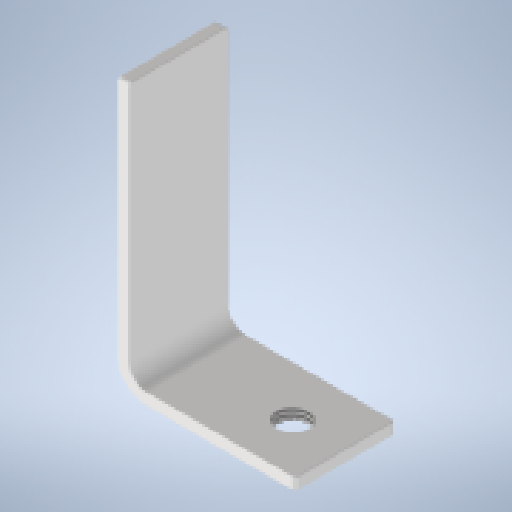
# Autodesk Inventor part: clampBaseBottom
Saved by Autodesk Inventor 2024.2 (Build 282272000, 272)
## iProperties
Created: 2024-05-25
Part Number: clampBaseBottom
Material: Generic
Document SubType Name: Modeling
Designer: user
Density: 1 g/cm^3
Appearance: Default
Author: user
Autodesk Inventor part; units mm, degrees
ref_plane "YZ Plane" through (0, 0, 0) normal (1, 0, 0) x (0, 1, 0)
ref_plane "XZ Plane" through (0, 0, 0) normal (0, 1, 0) x (-1, 0, 0)
ref_plane "XY Plane" through (0, 0, 0) normal (0, 0, 1) x (1, 0, 0)
sketch "Sketch1" plane through (0, 0, 0) normal (0, 0, 1) x (1, 0, 0)
  line L0 (0, 0) -> (-37, 0)
  line L1 (-43, 6) -> (-43, 66)
  arc A0 (-43, 6) -> (-37, 0) centre (-37, 6) ccw
  point P0 (-43, 0)
  dimension "d0" = 43
  dimension "d1" = 66
  dimension "d2" = 6
  constraints: 4 end point, 2 point on circle, 2 point on line, 2 tangent, 1 centre point, 1 horizontal, 1 vertical
  measures "d0" distance of L0.start point (-43, 0)
  measures "d1" distance of point (-43, 0) L1.end
  measures "d2" radius of A0
sketch "Sketch2" plane through (0, 0, 0) normal (1, 0, 0) x (0, 1, 0)
  line L0 (-1.5, -12.5) -> (1.5, -12.5)
  line L1 (1.5, -12.5) -> (1.5, 12.5)
  line L2 (1.5, 12.5) -> (-1.5, 12.5)
  line L3 (-1.5, 12.5) -> (-1.5, -12.5)
  line L4 (-1.5, -12.5) -> (1.5, 12.5) construction
  line L5 (1.5, -12.5) -> (-1.5, 12.5) construction
  point P0 (0, 0)
  dimension "d3" = 3
  dimension "d4" = 25
  constraints: 12 end point, 2 midpoint, 2 parallel, 1 horizontal, 1 perpendicular
  measures "d3" distance of L2.end L1.end
  measures "d4" distance of L1.end L0.end
sweep "Sweep1" add profiles "Sketch2" path "Sketch1" path curves L0 A0 L1
sketch "Sketch3" plane through (0, 1.5, 12.5) normal (0, 1, 0) x (1, 0, 0)
  circle A0 centre (-13, 12.5) radius 4
  line L0 (0, 25) -> (0, 0) projected
  point P0 (0, 12.5)
  point P1 (0, 12.5)
  point P2 (0, 12.5)
  dimension "d7" = 8
  dimension "d8" = 13
  constraints: 2 midpoint, 1 centre point, 1 horizontal alignment
  measures "d7" diameter of A0
  measures "d8" distance of point (0, 12.5) A0.centre
extrude "Extrusion1" cut sketch "Sketch3" against normal through all
thread "Thread1"
fillet "Fillet1" radius 1 4 edges at (-43, 66, 12.5) (0, 0, 12.5) (0, 0, -12.5) (-43, 66, -12.5)
fillet "Fillet2" radius 0.3 24 edges at (-44.5, 65.7071, 12.2071) (-44.5, 66, 0) (-44.5, 65.7071, -12.2071) (-44.5, 35.5, -12.5) (-42.3033, 0.6967, -12.5) (-19, -1.5, -12.5) (-0.2929, -1.5, -12.2071) (0, -1.5, 0) (-0.2929, -1.5, 12.2071) (-19, -1.5, 12.5) (-42.3033, 0.6967, 12.5) (-44.5, 35.5, 12.5) (-41.5, 65.7071, 12.2071) (-41.5, 66, 0) (-41.5, 65.7071, -12.2071) (-41.5, 35.5, -12.5) (-40.182, 2.818, -12.5) (-19, 1.5, -12.5) (-0.2929, 1.5, -12.2071) (0, 1.5, 0) (-0.2929, 1.5, 12.2071) (-19, 1.5, 12.5) (-40.182, 2.818, 12.5) (-41.5, 35.5, 12.5)
body "Solid1"
